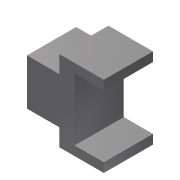
# Autodesk Inventor part: GARFO
Saved by Autodesk Inventor 2015 (Build 190159000, 159)
## iProperties
Created: 2016-08-09
Part Number: GARFO
Material: Aluminium AW-7020
Document SubType Name: Modeling
Designer: EriveltonDell
Density: 2.78 g/cm^3
Appearance: Stainless - Brushed
Mass: 1234.07 g
Surface Area: 731.335 cm^2
Volume: 443.911 cm^3
Author: EriveltonDell
Autodesk Inventor part; units mm, degrees
ref_plane "YZ Plane" through (0, 0, 0) normal (1, 0, 0) x (0, 1, 0)
ref_plane "XZ Plane" through (0, 0, 0) normal (0, 1, 0) x (-1, 0, 0)
ref_plane "XY Plane" through (0, 0, 0) normal (0, 0, 1) x (1, 0, 0)
sketch "Sketch5" plane through (0, 0, 0) normal (0, 1, 0) x (-1, 0, 0)
  line L0 (0, 0) -> (29, 0)
  line L1 (29, 0) -> (29, 52.5)
  line L2 (29, 52.5) -> (0, 52.5)
  line L3 (0, 0) -> (0, 6)
  line L4 (0, 6) -> (19, 6)
  line L5 (19, 6) -> (19, 46.5)
  line L6 (19, 46.5) -> (0, 46.5)
  line L7 (0, 52.5) -> (0, 46.5)
  line L8 (0, 6) -> (0, 0)
  dimension "d96" = 29
  dimension "d97" = 52.5
  dimension "d98" = 6
  dimension "d99" = 19
  dimension "d101" = 40.5
  constraints: 18 end point, 4 perpendicular, 3 parallel, 1 horizontal, 1 vertical
  measures "d96" distance of L2.end L1.end
  measures "d97" distance of L1.end L0.end
  measures "d98" distance of L0.start L3.end
  measures "d99" distance of L3.end L4.end
  measures "d101" distance of L4.end L5.end
extrude "Extrusion3" add sketch "Sketch5" along normal blind 32
sketch "Sketch6" plane through (-29, 0, 0) normal (-1, 0, 0) x (0, 0, 1)
  line L0 (26.25, 32) -> (41.25, 32)
  line L1 (41.25, 32) -> (41.25, 0)
  line L2 (41.25, 0) -> (11.25, 0)
  line L3 (11.25, 0) -> (11.25, 32)
  line L4 (11.25, 32) -> (26.25, 32)
  line L5 (0, 0) -> (52.5, 0) projected
  line L6 (0, 0) -> (0, 32) projected
  dimension "d106" = 15
  dimension "d107" = 32
  dimension "d108" = 30
  dimension "d109" = 32
  dimension "d110" = 0
  dimension "d111" = 11.25
  constraints: 10 end point, 1 perpendicular, 1 point on line
  measures "d106" distance of L0.start L0.end
  measures "d107" distance of L0.end L1.end
  measures "d108" distance of L1.end L2.end
  measures "d109" distance of L2.end L3.end
  measures "d110" distance between parallel lines of L2 L5
  measures "d111" distance between parallel lines of L3 L6
extrude "Extrusion4" add sketch "Sketch6" along normal blind 21
hole "Hole8" at (-50, 15, 26.25) direction (1, 0, 0) diameter 19 depth 15 tip angle 118
body "Solid3"
